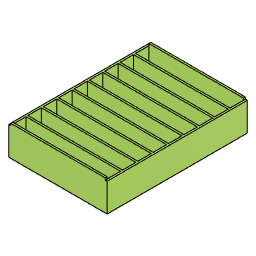
Dessicant Tray v4 (Autodesk Fusion 360 design; units mm, degrees)
Autodesk Fusion 360 part; units mm, degrees
sketch "Sketch2" plane through (0, 0, 0) normal (0, 1, 0) x (1, 0, 0)
  line L0 (76.2, 108.5) -> (-76.2, 108.5)
  line L1 (-76.2, 108.5) -> (-76.2, -108.5)
  line L2 (-76.2, -108.5) -> (76.2, -108.5)
  line L3 (76.2, -108.5) -> (76.2, 108.5)
  line L4 (76.2, 108.5) -> (-76.2, -108.5) construction
  line L5 (-76.2, 108.5) -> (76.2, -108.5) construction
  dimension "d14" = 152.4
  dimension "d15" = 217
  constraint horizontal L0
  constraint perpendicular L0 L1
  constraint parallel L0 L2
  constraint parallel L1 L3
  constraint coincident L4 origin
  constraint coincident L5 origin
  measures "d14" distance of L1.end L2.end
  measures "d15" distance of L0.end L1.end
extrude "Extrude1" add sketch "Sketch2" against normal blind 3
sketch "Sketch1" plane through (0, 0, 0) normal (0, 1, 0) x (1, 0, 0)
  line L0 (-73.2, -108.5) -> (-76.2, -108.5)
  line L1 (-76.2, -108.5) -> (-76.2, 108.5)
  line L2 (-76.2, 108.5) -> (-73.2, 108.5)
  line L3 (-73.2, 108.5) -> (-73.2, -108.5)
  line L4 (-73.2, -108.5) -> (-76.2, 108.5) construction
  line L5 (-76.2, -108.5) -> (-73.2, 108.5) construction
  line L6 (0, 0) -> (195.5563, 0) construction
  line L7 (73.2, 108.5) -> (76.2, 108.5)
  line L8 (76.2, 108.5) -> (76.2, -108.5)
  line L9 (76.2, -108.5) -> (73.2, -108.5)
  line L10 (73.2, -108.5) -> (73.2, 108.5)
  line L11 (-73.2, 108.5) -> (73.2, 108.5)
  line L12 (73.2, 108.5) -> (73.2, 105.5)
  line L13 (73.2, 105.5) -> (-73.2, 105.5)
  line L14 (-73.2, 105.5) -> (-73.2, 108.5)
  line L15 (73.2, 81.7222) -> (-73.2, 81.7222)
  line L16 (-73.2, 84.7222) -> (73.2, 84.7222)
  line L17 (73.2, 57.9444) -> (-73.2, 57.9444)
  line L18 (-73.2, 60.9444) -> (73.2, 60.9444)
  line L19 (73.2, 34.1667) -> (-73.2, 34.1667)
  line L20 (-73.2, 37.1667) -> (73.2, 37.1667)
  line L21 (73.2, 10.3889) -> (-73.2, 10.3889)
  line L22 (-73.2, 13.3889) -> (73.2, 13.3889)
  line L23 (73.2, -13.3889) -> (-73.2, -13.3889)
  line L24 (-73.2, -10.3889) -> (73.2, -10.3889)
  line L25 (73.2, -37.1667) -> (-73.2, -37.1667)
  line L26 (-73.2, -34.1667) -> (73.2, -34.1667)
  line L27 (73.2, -60.9444) -> (-73.2, -60.9444)
  line L28 (-73.2, -57.9444) -> (73.2, -57.9444)
  line L29 (73.2, -84.7222) -> (-73.2, -84.7222)
  line L30 (-73.2, -81.7222) -> (73.2, -81.7222)
  line L31 (73.2, -108.5) -> (-73.2, -108.5)
  line L32 (-73.2, -105.5) -> (73.2, -105.5)
  point P0 (-74.7, 0)
  dimension "d1" = 217
  dimension "d6" = 3
  dimension "d8" = 152.4
  dimension "d9" = 3
  dimension "d12" = 0
  dimension "d21" = 76.2
  constraint horizontal L0
  constraint perpendicular L0 L1
  constraint parallel L0 L2
  constraint parallel L1 L3
  constraint coincident L4 P0
  constraint coincident L5 P0
  constraint coincident L6.start origin
  constraint horizontal L6
  constraint coincident P0 L6
  constraint horizontal L7
  constraint vertical L8
  constraint horizontal L9
  constraint vertical L10
  constraint collinear L2 L7
  constraint collinear L0 L9
  constraint equal L2 L7
  constraint horizontal L11
  constraint vertical L12
  constraint horizontal L13
  constraint vertical L14
  constraint collinear L3 L14
  constraint collinear L10 L12
  constraint collinear L2 L11
  measures "d1" distance of L0.end L1.end
  measures "d6" distance of L1.end L2.end
  measures "d8" distance of L0.end L8.end
  measures "d9" distance of L11 L13
  measures "d21" distance of L6.start L1
extrude "Extrude2" add sketch "Sketch1" along normal blind 42 contours L0 L1 L2 L3 L14 | L7 L8 L9 L10 L12 | L3 L10 L29 L30 | L3 L10 L27 L28 | L3 L10 L15 L16 | L3 L10 L25 L26 | L3 L10 L17 L18 | L3 L10 L23 L24 | L3 L10 L19 L20 | L3 L10 L21 L22
extrude "Extrude3" add sketch "Sketch1" along normal blind 45 contours L3 L10 L31 L32 | L3 L10 L11 L12 L13 L14
chamfer "Chamfer1" distance 1 angle 45 4 edges at (0, -3, -108.5) (-76.2, -3, 0) (76.2, -3, 0) (0, -3, 108.5) measured on face at (-25.4, -3, -36.1667) measured on face at (-25.4, -3, -36.1667) measured on face at (-25.4, -3, -36.1667) measured on face at (-25.4, -3, -36.1667)
equation "d1 = Length"
equation "Length = 217 mm"
equation "Width = 6 in"
equation "Wall_Thickness = 3 mm"
equation "Number_of_Ribs = 10"
equation "d6 = Wall_Thickness"
equation "d8 = Width"
equation "d9 = Wall_Thickness"
equation "d13 = -( Length - Wall_Thickness )"
equation "d14 = Width"
equation "d15 = Length"
equation "Height = 45 mm"
equation "d19 = Height - Wall_Thickness"
equation "d21 = Width / 2"
equation "BaseWallThickness_1 = 3 mm"
equation "BearingHolderHeight_1 = 20 mm"
equation "BearingHolderDistance_1 = 80 mm"
equation "BearingHolderDiameter_1 = 7.8 mm"
equation "BaseInsideWidth_1 = 70 mm"
equation "BaseLength_1 = 190 mm"
equation "BaseWallHeight_1 = 100 mm"
equation "d22 = Height"
equation "BaseWallThickness_2 = 3 mm"
equation "BearingHolderHeight_2 = 20 mm"
equation "BearingHolderDistance_2 = 80 mm"
equation "BearingHolderDiameter_2 = 7.8 mm"
equation "BaseInsideWidth_2 = 70 mm"
equation "BaseLength_2 = 190 mm"
equation "BaseWallHeight_2 = 100 mm"
